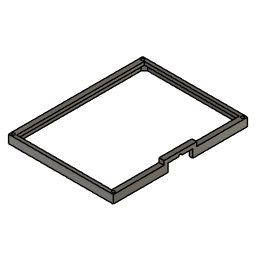
cover_rain (Autodesk Fusion 360 design; units mm, degrees)
Autodesk Fusion 360 part; units mm, degrees
sketch "Sketch1" plane through (0, 0, 0) normal (0, 0, 1) x (1, 0, 0)
  line L0 (58, 78) -> (-58, 78)
  line L1 (-58, 78) -> (-58, -78)
  line L2 (-58, -78) -> (58, -78)
  line L3 (58, -78) -> (58, 78)
  line L4 (58, 78) -> (-58, -78) construction
  line L5 (-58, 78) -> (58, -78) construction
  circle A0 centre (-61, 79) radius 1.75
  line L6 (0, 2.5) -> (0, 20)
  circle A1 centre (61, 79) radius 1.75
  line L7 (20, 0) -> (2.5, 0)
  circle A2 centre (61, -79) radius 1.75
  circle A3 centre (-61, -79) radius 1.75
  line L8 (64, 82) -> (-64, 82)
  line L9 (-64, 82) -> (-64, -82)
  line L10 (-64, -82) -> (64, -82)
  line L11 (64, -82) -> (64, 82)
  line L12 (64, 82) -> (-64, -82) construction
  line L13 (-64, 82) -> (64, -82) construction
  dimension "d1" = 116
  dimension "d2" = 156
  dimension "d3" = 3.5
  dimension "d4" = 3
  dimension "d5" = 1
  dimension "d6" = 3
  dimension "d7" = 3
  constraint horizontal L0
  constraint perpendicular L0 L1
  constraint parallel L0 L2
  constraint parallel L1 L3
  constraint coincident L4 origin
  constraint coincident L5 origin
  constraint symmetric A0 L6 A1
  constraint symmetric A0 L7 A3
  constraint symmetric A1 L7 A2
  constraint horizontal L8
  constraint perpendicular L8 L9
  constraint parallel L8 L10
  constraint parallel L9 L11
  constraint coincident L12 origin
  constraint coincident L13 origin
  measures "d1" distance of L1.end L2.end
  measures "d2" distance of L0.end L1.end
  measures "d3" diameter of A0
  measures "d4" horizontal distance of L0.end A0.centre
  measures "d5" vertical distance of L0.end A0.centre
  measures "d6" distance of A0.centre L8
  measures "d7" distance of A0.centre L9
extrude "Extrude1" add sketch "Sketch1" along normal blind 10
sketch "Sketch2" plane through (0, 0, 0) normal (0, 0, 1) x (-1, 0, 0)
  line L0 (-58, -78) -> (-58, 78)
  line L1 (-58, 78) -> (58, 78)
  line L2 (58, 78) -> (58, -78)
  line L3 (58, -78) -> (-58, -78)
  circle A0 centre (-61, 79) radius 1.5
  circle A1 centre (-61, -79) radius 1.5
  circle A2 centre (61, 79) radius 1.5
  circle A3 centre (61, -79) radius 1.5
  line L4 (-64, 82) -> (-64, -82)
  line L5 (-64, -82) -> (64, -82)
  line L6 (64, -82) -> (64, 82)
  line L7 (64, 82) -> (-64, 82)
  line L8 (-60, 80) -> (60, 80)
  line L9 (60, 80) -> (60, -80)
  line L10 (60, -80) -> (-60, -80)
  line L11 (-60, -80) -> (-60, 80)
  line L12 (56, -80) -> (60, -76)
  line L13 (0, -2.5) -> (0, -20)
  line L14 (-56, -80) -> (-60, -76)
  line L15 (-20, 0) -> (-2.5, 0)
  line L16 (-56, 80) -> (-60, 76)
  line L17 (56, 80) -> (60, 76)
  line L18 (-58, 78) -> (-58, -78)
  line L19 (-58, -78) -> (58, -78)
  line L20 (58, -78) -> (58, 78)
  line L21 (58, 78) -> (-58, 78)
  circle A4 centre (-61, 79) radius 1.75
  circle A5 centre (-61, -79) radius 1.75
  circle A6 centre (61, 79) radius 1.75
  circle A7 centre (61, -79) radius 1.75
  line L22 (-64, -82) -> (-64, 82)
  line L23 (-64, 82) -> (64, 82)
  line L24 (64, 82) -> (64, -82)
  line L25 (64, -82) -> (-64, -82)
  dimension "d10" = -2
  dimension "d11" = 45
  constraint coincident L10 L12.start
  constraint coincident L9 L12.end
  constraint coincident L2.end L12
  constraint symmetric L12.start L13 L14.start
  constraint symmetric L12.end L13 L14.end
  constraint symmetric L12.start L15 L17.start
  constraint symmetric L12.end L15 L17.end
  constraint symmetric L14.start L15 L16.start
  constraint symmetric L14.end L15 L16.end
  measures "d11" angle of L3 L12
extrude "Extrude2" cut sketch "Sketch2" along normal blind 6 contours L0 L11 L14 L16 L18 | L3 L10 L12 L14 L19 | L1 L8 L16 L17 L21 | L2 L9 L12 L17 L20
sketch "Sketch3" plane through (0, 0, 0) normal (0, 0, 1) x (1, 0, 0)
  line L0 (58, 15) -> (64, 15)
  line L1 (64, 15) -> (64, -15)
  line L2 (64, -15) -> (58, -15)
  line L3 (58, -15) -> (58, 15)
  line L4 (64, -82) -> (64, 82)
  line L5 (58, -78) -> (58, 78)
  line L6 (58, 15) -> (64, 15)
  line L7 (64, 15) -> (64, 20)
  line L8 (64, 20) -> (58, 20)
  line L9 (58, 20) -> (58, 15)
  line L10 (58, -15) -> (64, -15)
  line L11 (64, -15) -> (64, -20)
  line L12 (64, -20) -> (58, -20)
  line L13 (58, -20) -> (58, -15)
  point P0 (58, 0)
  dimension "d14" = 30
  dimension "d15" = 5
  dimension "d16" = 5
  constraint horizontal L0
  constraint vertical L1
  constraint horizontal L2
  constraint vertical L3
  constraint midpoint L3 P0
  constraint horizontal origin P0
  constraint collinear L1 L4
  constraint collinear L3 L5
  constraint horizontal L6
  constraint vertical L7
  constraint horizontal L8
  constraint vertical L9
  constraint horizontal L10
  constraint vertical L11
  constraint horizontal L12
  constraint vertical L13
  measures "d14" distance of L0 L2
  measures "d15" distance of L0.start L8.end
  measures "d16" distance of L2.end L12.end
extrude "Extrude3" add sketch "Sketch3" along normal blind 15
extrude "Extrude4" cut sketch "Sketch3" along normal blind 10 contours L0 L1 L2 L3 L4 L5 L6 L10
sketch "Sketch4" plane through (58, 0, 0) normal (-1, 0, 0) x (0, -1, 0)
  line L0 (-15, 0) -> (-15, 10)
  line L1 (-15, 10) -> (15, 10)
  line L2 (15, 10) -> (15, 0)
  line L3 (15, 0) -> (20, 0)
  line L4 (78, 6) -> (78, 10)
  line L5 (20, 6) -> (78, 6)
  line L6 (20, 0) -> (20, 6)
  line L7 (20, 15) -> (-20, 15)
  line L8 (-20, 15) -> (-20, 10)
  line L9 (-78, 10) -> (-78, 6)
  circle A0 centre (0, 10) radius 2
  line L10 (78, 10) -> (20, 10)
  line L11 (20, 10) -> (20, 15)
  line L12 (-20, 10) -> (-78, 10)
  line L13 (-78, 6) -> (-20, 6)
  line L14 (-20, 6) -> (-20, 0)
  line L15 (-20, 0) -> (-15, 0)
  constraint midpoint L1 A0.centre
extrude "Extrude5" cut sketch "Sketch4" against normal blind 6 contours L1 A0 picked at (0.4887, 10.4534)
sketch "Sketch6" plane through (58, 0, 0) normal (-1, 0, 0) x (0, -1, 0)
  arc A0 (2, 10) -> (-2, 10) centre (0, 10) ccw
  line L0 (2, 10) -> (15, 10)
  line L1 (15, 10) -> (15, 0)
  line L2 (15, 0) -> (20, 0)
  line L3 (20, 0) -> (20, 6)
  line L4 (20, 6) -> (78, 6)
  line L5 (78, 6) -> (78, 10)
  line L6 (78, 10) -> (20, 10)
  line L7 (20, 10) -> (20, 15)
  line L8 (20, 15) -> (-20, 15)
  line L9 (-20, 15) -> (-20, 10)
  line L10 (-20, 10) -> (-78, 10)
  line L11 (-78, 10) -> (-78, 6)
  line L12 (-78, 6) -> (-20, 6)
  line L13 (-20, 6) -> (-20, 0)
  line L14 (-20, 0) -> (-15, 0)
  line L15 (-15, 0) -> (-15, 10)
  line L16 (-15, 10) -> (-2, 10)
  line L17 (-20, 6) -> (-18, 6)
  line L18 (-18, 6) -> (-18, 13)
  line L19 (-18, 13) -> (18, 13)
  line L20 (18, 13) -> (18, 6)
  line L21 (18, 6) -> (20, 6)
  dimension "d26" = 3
  dimension "d27" = 3
  dimension "d28" = 3
  constraint coincident L12.end L13.start
  constraint perpendicular L13 L17
  constraint perpendicular L17 L18
  constraint perpendicular L18 L19
  constraint perpendicular L19 L20
  constraint coincident L3.end L4.start
  measures "d26" distance of L15 L18
  measures "d27" distance of L16 L19
  measures "d28" distance of L1 L19.end
extrude "Extrude7" cut sketch "Sketch6" against normal blind 2 contours A0 L0 L1 L2 L3 L13 L14 L15 L16 L17 L18 L19 L20 L21
